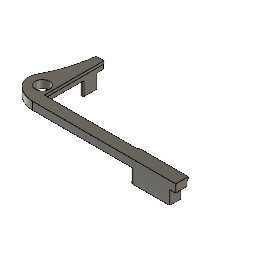
antenna mount (Autodesk Fusion 360 design; units mm, degrees)
Autodesk Fusion 360 part; units mm, degrees
sketch "Skizze1" plane through (0, 0, 0) normal (0, 0, 1) x (1, 0, 0)
  circle A0 centre (0, 0) radius 1.5
  line L0 (0, 0) -> (0, 11.2) construction
  line L1 (0, 0) -> (32.75, 0) construction
  circle A1 centre (0, 0) radius 3.1
  line L2 (1.9, -1.6) -> (32.65, -1.6)
  line L3 (32.65, -1.6) -> (32.65, -4.0474)
  line L4 (1.9, -1.6) -> (1.9, 11.2)
  line L5 (1.9, 11.2) -> (0.3052, 11.2)
  arc A2 (-2.7333, 1.4626) -> (0.3052, 11.2) centre (-26.6828, 14.2787) ccw
  line L6 (0.3052, 11.2) -> (0, 11.2) construction
  arc A3 (-2.4759, -1.8655) -> (1.9, -4.0474) centre (1.9, 1.4316) ccw
  line L7 (1.9, -4.0474) -> (32.65, -4.0474)
  line L8 (1.2, 2.8583) -> (1.2, 11.2)
  line L9 (1.2, 10) -> (1.9, 10)
  arc A4 (1.9, 6.7372) -> (1.2, 6.8964) centre (0, 0) ccw
  line L10 (1.5, 0) -> (1.9, 0)
  line L11 (31.35, -4.0474) -> (31.35, -1.6)
  line L12 (22.6001, -4.0474) -> (22.6001, -1.6)
  line L13 (30.5501, -3.2474) -> (30.5501, -2.4)
  line L14 (1.2, 9.2) -> (1.9, 9.2)
  line L15 (23.3999, -2.4) -> (30.5501, -2.4)
  line L16 (23.3999, -3.2474) -> (30.5501, -3.2474)
  line L17 (23.3999, -2.4) -> (23.3999, -3.2474)
  dimension "d1" = 3
  dimension "d2" = 11.2
  dimension "d3" = 32.75
  dimension "d4" = 1.6
  dimension "d8" = 1.2
  dimension "d9" = 1.2
  dimension "d14" = 0.4
  dimension "d15" = 1.3
  dimension "d16" = 0.1
  dimension "d26" = 7
  dimension "d41" = 0.8
  dimension "d42" = 0.8
  dimension "d43" = 7.95
  dimension "d48" = 1.6
  constraint coincident A0.centre L0.start
  constraint vertical L0
  constraint perpendicular L0 L1
  constraint horizontal L2
  constraint perpendicular L2 L3
  constraint coincident L2 L4.start
  constraint perpendicular L2 L4
  constraint perpendicular L4 L5
  constraint coincident A1 A2.start
  constraint tangent A1 A2
  constraint horizontal L6
  constraint tangent A1 A3
  constraint coincident A1 A3.start
  constraint perpendicular L3 L7
  constraint tangent A3 L7
  constraint coincident L4 A3.centre
  constraint coincident A1 L8.start
  constraint coincident L5 L8.end
  constraint perpendicular L5 L8
  constraint coincident L8 L9.start
  constraint coincident L4 L9.end
  constraint perpendicular L4 L9
  constraint coincident L8 A4.end
  constraint coincident A0 L10.start
  constraint coincident L1 L10.start
  constraint coincident L4 L10.end
  constraint coincident L1 L10.end
  constraint coincident L7 L11.start
  constraint coincident L2 L11.end
  constraint perpendicular L2 L11
  constraint coincident L7 L12.start
  constraint coincident L2 L12.end
  constraint perpendicular L2 L12
  constraint concentric A0 A4
  constraint coincident L13 L15.end
  constraint perpendicular L13 L15
  constraint coincident L13 L16.end
  constraint perpendicular L13 L16
  constraint parallel L9 L14
  constraint coincident L4 A4.start
  constraint parallel L11 L13
  constraint perpendicular L16 L17
  constraint coincident L4 L14.end
  measures "d1" diameter of A0
  measures "d2" distance of A0.centre L0.end
  measures "d3" distance of A0.centre L1.end
  measures "d8" distance of L0 L8
  measures "d9" distance of L5 L9
  measures "d14" distance of L10.start L10.end
  measures "d15" distance of L3 L11
  measures "d16" distance of L1.end L3
  measures "d26" radius of A4
  measures "d41" distance of L7 L16
  measures "d42" distance of L2 L15
  measures "d43" distance of L12 L13
  measures "d48" vertical distance of A0.centre L2.start
extrude "Extrusion1" add sketch "Skizze1" along normal blind 1.1 contours A1 L2 L4 | A1 L4 L8 A4 | A1 L5 A2 L8 | L4 L8 A4 L14 | A1 L2 A3 L7 L12 | L4 L8 L9 L14 | L4 L5 L8 L9 | L2 L7 L11 L12 | L2 L3 L7 L11 | L13 L15 L16 L17 picked at (1.3516, -1.8875)
extrude "Extrusion2" add sketch "Skizze1" against normal blind 3 contours L4 L8 A4 L14 | L4 L8 L9 L14 | L2 L7 L11 L12
fillet "Abrundung1" radius 0.8 2 edges at (22.6001, -4.0474, -1.5) (22.6001, -1.6, -1.5)
fillet "Abrundung1" radius 0.4 4 edges at (23.3999, -3.2474, -1.5) (23.3999, -2.4, -1.5) (30.5501, -2.4, -1.5) (30.5501, -3.2474, -1.5)
fillet "Abrundung1" radius 0.2 4 edges at (1.2, 6.8964, -1.5) (1.9, 6.7372, -1.5) (1.2, 10, -1.5) (1.9, 10, -1.5)
sketch "Skizze2" plane through (0, 0, 1.1) normal (0, 0, 1) x (-1, 0, 0)
  circle A0 centre (0, 0) radius 1.5
  arc A1 (2.7333, -1.4626) -> (2.4759, 1.8655) centre (0, 0) ccw
  arc A2 (2.4759, 1.8655) -> (-1.9, 4.0474) centre (-1.9, -1.4316) ccw
  line L0 (-1.9, 4.0474) -> (-32.65, 4.0474)
  line L1 (-32.65, 4.0474) -> (-32.65, 1.6)
  line L2 (-32.65, 1.6) -> (-1.9, 1.6)
  line L3 (-1.9, 1.6) -> (-1.9, -11.2)
  line L4 (-1.9, -11.2) -> (-0.3052, -11.2)
  arc A3 (2.7333, -1.4626) -> (-0.3052, -11.2) centre (26.6828, -14.2787) ccw
  line L5 (-32.65, 1.3) -> (-2.05, 1.3)
  line L6 (-2.05, 1.3) -> (-2.05, -11.2)
  line L7 (-1.9, -11.2) -> (-2.05, -11.2)
  line L8 (-32.65, 1.3) -> (-32.65, 1.6)
  line L9 (-22.05, 1.3) -> (-22.05, 1.6)
  line L10 (-2.05, 1.3) -> (-2.05, 1.6)
  dimension "d40" = 20
  dimension "d46" = 0.3
  dimension "d47" = 0.15
  constraint coincident L3.end L4.start
  constraint perpendicular L6 L7
  constraint coincident L1.end L2.start
  constraint perpendicular L2 L8
  constraint coincident L5 L9.start
  constraint coincident L2 L9.end
  constraint perpendicular L2 L9
  constraint coincident L2 L10.end
  constraint perpendicular L2 L10
  constraint parallel L2 L5
  constraint parallel L3 L6
  measures "d40" distance of L9.end L10.end
  measures "d46" distance of L2 L5
  measures "d47" distance of L3 L6
extrude "Extrusion3" add sketch "Skizze2" along normal blind 0.6 contours A1 A2 L0 L1 L2 L3 L4 A3 | L2 L3 L6 L7 L10 | L2 L5 L8 L9
